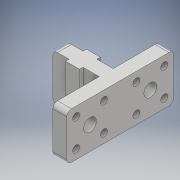
# Autodesk Inventor part: Estrutura - Cabos
Saved by Autodesk Inventor 2017 (Build 210142000, 142)
## iProperties
Created: 2020-08-30
Part Number: Estrutura - Cabos
Material: Generic
Document SubType Name: Modeling
Designer: ale
Density: 1 g/cm^3
Appearance: Default
Author: ale
Autodesk Inventor part; units mm, degrees
ref_plane "YZ Plane" through (0, 0, 0) normal (1, 0, 0) x (0, 1, 0)
ref_plane "XZ Plane" through (0, 0, 0) normal (0, 1, 0) x (-1, 0, 0)
sketch "Sketch1" plane through (0, 0, 0) normal (0, 0, 1) x (1, 0, 0)
  line L0 (0, 0) -> (0, -20)
  line L1 (0, 0) -> (-20, 0)
  line L2 (-20, 6) -> (0, 6)
  line L3 (6, 26) -> (6, -20)
  line L4 (-20, 0) -> (-20, 6)
  line L5 (0, -20) -> (6, -20)
  line L6 (0, 6) -> (0, 26)
  line L7 (0, 26) -> (6, 26)
  dimension "d0" = 20
  dimension "d1" = 20
  dimension "d2" = 6
  dimension "d3" = 26
  dimension "d4" = 6
  dimension "d5" = 46
  constraints: 16 end point, 4 perpendicular, 2 vertical, 1 horizontal
  measures "d0" distance of L0.start L0.end
  measures "d1" distance of L0.start L1.end
  measures "d2" distance between parallel lines of L1 L2
  measures "d3" distance of L0.start L6.end
  measures "d4" distance of L3.start L6.end
  measures "d5" distance between parallel lines of L7 L5
extrude "Extrusion1" add sketch "Sketch1" along normal blind 20
sketch "Sketch2" plane through (-20, 0, 0) normal (0, -1, 0) x (1, 0, 0)
  line L0 (0, 20) -> (20, 20) projected
  line L1 (7, 20) -> (7, 0)
  line L2 (7, 0) -> (13, 0)
  line L3 (0, 0) -> (20, 0) projected
  line L4 (13, 0) -> (13, 20)
  line L5 (13, 20) -> (7, 20)
  line L6 (0, 0) -> (0, 20) projected
  dimension "d8" = 6
  dimension "d9" = 7
  constraints: 8 end point, 2 perpendicular, 2 point on line, 1 vertical
  measures "d8" distance of L1.end L2.end
  measures "d9" distance between parallel lines of L6 L1
extrude "Extrusion2" add sketch "Sketch2" along normal blind 1.5 contours L0 L4 L2 L1
ref_plane "Work Plane1" through (-20, 3, 0) normal (0, -1, 0) x (1, 0, 0)
mirror "Mirror1" about plane through (-20, 3, 0) normal (0, -1, 0) of "Extrusion2"
sketch "Sketch3" plane through (6, -20, 0) normal (1, 0, 0) x (0, 0, -1)
  line L0 (0, 0) -> (-20, 0) projected
  line L1 (0, 0) -> (0, 46) projected
  line L2 (-20, 0) -> (-20, 46) projected
  line L3 (-20, 23) -> (0, 23)
  point P0 (0, 20)
  point P1 (-10, 10)
  point P2 (-10, 36)
  dimension "d13" = 10
  dimension "d14" = 10
  constraints: 2 end point, 2 midpoint, 1 symmetric about line
  measures "d13" distance from line of L0 point (-10, 10)
  measures "d14" distance from line of L1 point (-10, 10)
hole "Hole1" at (6, -10, 10) at (6, 16, 10) direction (-1, 0, 0) diameter 5.5 end through all
sketch "Sketch4" plane through (6, -20, 0) normal (1, 0, 0) x (0, 0, -1)
  line L0 (-20, 20) -> (-20, 0) projected
  line L1 (-20, 10) -> (0, 10)
  line L2 (0, 20) -> (0, 0) projected
  line L3 (0, 0) -> (-20, 0) projected
  line L4 (-10, 0) -> (-10, 29.1489)
  line L5 (-20, 0) -> (-20, 46) projected
  line L6 (-20, 23) -> (0, 23)
  line L7 (0, 26) -> (0, 20) projected
  point P0 (-16, 4)
  point P1 (-16, 16)
  point P2 (-4, 4)
  point P3 (-4, 16)
  point P4 (-16, 42)
  point P5 (-16, 30)
  point P6 (-4, 42)
  point P7 (-4, 30)
  dimension "d22" = 6
  dimension "d23" = 6
  constraints: 7 symmetric about line, 6 end point, 5 midpoint, 1 vertical
  measures "d22" distance from line of point (-16, 4) L1
  measures "d23" distance from line of point (-16, 4) L4
hole "Hole2" at (6, -16, 16) at (6, -4, 16) at (6, -16, 4) at (6, -4, 4) at (6, 22, 16) at (6, 10, 16) at (6, 10, 4) at (6, 22, 4) direction (-1, 0, 0) diameter 3 end through all
fillet "Fillet1" radius 2 6 edges at (3, -20, 20) (3, 26, 20) (3, 26, 0) (3, -20, 0) (-20, 3, 20) (-20, 3, 0)
body "Solid1"
